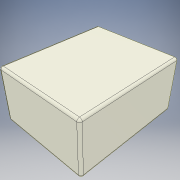
# Autodesk Inventor part: Button
Saved by Autodesk Inventor 2018 (Build 220112000, 112)
## iProperties
Created: 2021-02-07
Part Number: Button
Material: Všeobecné
Document SubType Name: Modeling
Designer: Jozko Mrkvicka
Density: 1 g/cm^3
Appearance: Výchozí
Author: Jozko Mrkvicka
Autodesk Inventor part; units mm, degrees
ref_plane "YZ Plane" through (0, 0, 0) normal (1, 0, 0) x (0, 1, 0)
ref_plane "XZ Plane" through (0, 0, 0) normal (0, 1, 0) x (-1, 0, 0)
ref_plane "XY Plane" through (0, 0, 0) normal (0, 0, 1) x (1, 0, 0)
sketch "Náčrt1" plane through (0, 0, 0) normal (0, 1, 0) x (-1, 0, 0)
  line L0 (0, 0) -> (9.525, 0)
  line L1 (9.525, 0) -> (9.525, -5.715)
  line L2 (9.525, -5.715) -> (0, -5.715)
  line L3 (0, -5.715) -> (0, 0)
  dimension "d0" = 9.525
  dimension "d1" = 5.715
  constraints: 8 end point, 2 parallel, 1 horizontal, 1 perpendicular
  measures "d0" distance of L1.end L2.end
  measures "d1" distance of L0.end L1.end
extrude "Vysunutí1" add sketch "Náčrt1" along normal blind 11.43
sketch "Náčrt2" plane through (0, 0, 0) normal (0, -1, 0) x (1, 0, 0)
  line L0 (-1.27, -4.445) -> (-1.27, -1.27)
  line L1 (-8.255, -1.27) -> (-8.255, -4.445)
  line L2 (-6.35, -4.445) -> (-3.175, -4.445)
  line L3 (-3.175, -1.27) -> (-6.35, -1.27)
  line L4 (-2.54, -1.27) -> (-2.54, -1.905)
  line L5 (-2.54, -1.905) -> (-3.175, -1.905)
  line L6 (-3.175, -1.905) -> (-3.175, -1.27)
  line L7 (-2.54, -4.445) -> (-2.54, -3.81)
  line L8 (-2.54, -3.81) -> (-3.175, -3.81)
  line L9 (-3.175, -3.81) -> (-3.175, -4.445)
  line L10 (-6.985, -4.445) -> (-6.985, -3.81)
  line L11 (-6.985, -3.81) -> (-6.35, -3.81)
  line L12 (-6.35, -3.81) -> (-6.35, -4.445)
  line L13 (-6.985, -1.27) -> (-6.985, -1.905)
  line L14 (-6.985, -1.905) -> (-6.35, -1.905)
  line L15 (-6.35, -1.905) -> (-6.35, -1.27)
  line L16 (-6.985, -1.27) -> (-8.255, -1.27)
  line L17 (-8.255, -4.445) -> (-6.985, -4.445)
  line L18 (-6.35, -4.445) -> (-3.175, -4.445)
  line L19 (-2.54, -4.445) -> (-1.27, -4.445)
  line L20 (-1.27, -1.27) -> (-2.54, -1.27)
  line L21 (-3.175, -1.27) -> (-6.35, -1.27)
  point P0 (-4.7625, -2.8575)
  constraints: 44 end point, 15 parallel, 4 horizontal, 4 point on line, 3 perpendicular
extrude "Vysunutí2" cut sketch "Náčrt2" against normal blind 9.525
fillet "Zaoblení1" radius 0.254 8 edges at (-4.7625, 11.43, 0) (-9.525, 5.715, 0) (-9.525, 11.43, -2.8575) (0, 11.43, -2.8575) (-4.7625, 11.43, -5.715) (-9.525, 5.715, -5.715) (0, 5.715, 0) (0, 5.715, -5.715)
